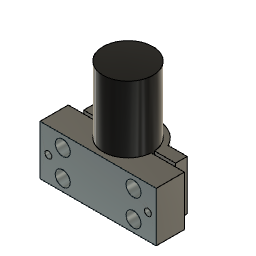
back_holder_thick (Autodesk Fusion 360 design; units mm, degrees)
Autodesk Fusion 360 part; units mm, degrees
note: some values were not read from the file. Set by a fixed rule: which sketch regions a step uses.
sketch "Sketch1" plane through (0, 0, 0) normal (0, 0, 1) x (1, 0, 0) in component "Pipe"
  circle A0 centre (0, 0) radius 15
  dimension "d1" = 30
  constraint coincident A0.centre origin
  measures "d1" diameter of A0
extrude "Extrude1" add sketch "Sketch1" along normal blind 70 makes body 1 in component "Pipe"
sketch "Sketch1 (2)" plane through (0, 0, 0) normal (0, 0, 1) x (1, 0, 0) in component "holder_under"
  circle A0 centre (0, 0) radius 15
  circle A1 centre (0, 0) radius 18
  line L0 (-17.9722, 1) -> (-27.6886, 1)
  line L1 (-27.6886, 1) -> (-27.6886, 8)
  line L2 (-27.6886, 8) -> (-12.6886, 8)
  line L3 (0, 0) -> (0, 15) construction
  line L4 (27.6886, 8) -> (12.6886, 8)
  line L5 (27.6886, 1) -> (27.6886, 8)
  line L6 (17.9722, 1) -> (27.6886, 1)
  line L7 (-17.9722, 1) -> (-14.9666, 1)
  line L8 (17.9722, 1) -> (14.9666, 1)
  dimension "d4" = 3
  dimension "d5" = 7
  dimension "d6" = 15
  dimension "d7" = 1
  constraint coincident A1 L0.start
  constraint horizontal L0
  constraint perpendicular L0 L1
  constraint coincident A0 L2.end
  constraint perpendicular L1 L2
  constraint coincident A0.centre A1.centre
  constraint coincident A0 L3.end
  constraint vertical L3
  constraint symmetric L0.start L3 L6.start
  constraint symmetric L0.end L3 L5.start
  constraint symmetric L1.end L3 L4.start
  constraint symmetric L2.end L3 L4.end
  constraint coincident A0 L7.end
  constraint parallel L0 L7
  constraint coincident A0 L8.end
  constraint parallel L6 L8
  measures "d5" distance of L0.end L1.end
  measures "d6" distance of L1.end L2.end
  measures "d7" distance of A0.centre L0
extrude "Extrude1'" add sketch "Sketch1 (2)" along normal blind 30 separate body contours A0 A1 L4 L8 | A0 A1 L2 L7 | A0 A1 L2 L4 | A1 L4 L5 L6 | A1 L0 L1 L2 makes body 2 in component "holder_under"
sketch "Sketch2" plane through (0, 1, 0) normal (0, -1, 0) x (1, 0, 0) in component "holder_under"
  line L0 (14.9666, 0) -> (27.6886, 0)
  line L1 (27.6886, 0) -> (27.6886, 30)
  line L2 (27.6886, 30) -> (14.9666, 30)
  line L3 (14.9666, 30) -> (14.9666, 0)
  line L4 (-21.3276, 30) -> (-21.3276, 0) construction
  line L5 (-27.6886, 30) -> (-14.9666, 30)
  line L6 (-14.9666, 0) -> (-27.6886, 0)
  line L7 (0, 0) -> (0, 30) construction
  line L8 (-14.9666, 30) -> (14.9666, 30)
  circle A0 centre (-21.3276, 23) radius 2.075
  circle A1 centre (-21.3276, 7) radius 2.075
  circle A2 centre (21.3276, 23) radius 2.075
  circle A3 centre (21.3276, 7) radius 2.075
  dimension "d10" = 4.15
  dimension "d11" = 4.15
  dimension "d12" = 7
  dimension "d13" = 7
  constraint vertical L4
  constraint coincident L4.start L5
  constraint coincident L4.end L6
  constraint midpoint L4.start L5
  constraint coincident L7.start origin
  constraint perpendicular L5 L7
  constraint coincident L7.end L8
  constraint coincident L4 A0.centre
  constraint coincident L4 A1.centre
  constraint symmetric L7 A0 A2
  constraint symmetric L7 A1 A3
  measures "d10" diameter of A0
  measures "d11" diameter of A1
  measures "d12" distance of L6 A1.centre
  measures "d13" distance of L5 A0.centre
extrude "Extrude2" cut sketch "Sketch2" against normal up to surface (7 mm away) contours A0 | A1 | A2 | A3 bodies 2 in component "holder_under"
sketch "Sketch1 (3)" plane through (0, 0, 0) normal (0, 0, 1) x (1, 0, 0) in component "holder_top"
  circle A0 centre (0, 0) radius 15
  circle A1 centre (0, 0) radius 18
  line L0 (-17.9722, -1) -> (-35, -1)
  line L1 (-35, -1) -> (-35, -18)
  line L2 (-35, -18) -> (0, -18)
  line L3 (0, 0) -> (0, -18) construction
  line L4 (35, -1) -> (35, -18)
  line L5 (35, -18) -> (0, -18)
  line L6 (17.9722, -1) -> (35, -1)
  line L7 (17.9722, -1) -> (14.9666, -1)
  line L8 (-17.9722, -1) -> (-14.9666, -1)
  dimension "d16" = 3
  dimension "d17" = 1
  dimension "d18" = 35
  constraint coincident A1 L0.start
  constraint horizontal L0
  constraint perpendicular L0 L1
  constraint perpendicular L1 L2
  constraint coincident A1 L2.end
  constraint tangent A1 L2
  constraint coincident A0.centre A1.centre
  constraint symmetric L0.start L3 L6.start
  constraint symmetric L0.end L3 L4.start
  constraint symmetric L1.end L3 L4.end
  constraint symmetric L2.end L3 L5.end
  constraint coincident A0 L7.end
  constraint parallel L6 L7
  constraint coincident A0 L8.end
  constraint parallel L0 L8
  measures "d17" distance of A0.centre L0
  measures "d18" distance of L1.end L2.end
extrude "Extrude1''" add sketch "Sketch1 (3)" along normal up to surface (30 mm away) separate body contours A0 A1 L7 L8 | A1 L0 L1 L2 | A1 L4 L5 L6 picked at (-1.1817, -16.9303) makes body 3 in component "holder_top"
sketch "Sketch2 (2)" plane through (0, -1, 0) normal (0, 1, 0) x (-1, 0, 0) in component "holder_top"
  line L0 (-14.9666, 30) -> (-35, 30)
  line L1 (-35, 30) -> (-35, 0)
  line L2 (-35, 0) -> (-14.9666, 0)
  line L3 (-14.9666, 0) -> (-14.9666, 30)
  circle A0 centre (-21.3276, 23) radius 2.075
  circle A1 centre (-21.3276, 7) radius 2.075
  circle A2 centre (21.3276, 7) radius 2.075
  circle A3 centre (21.3276, 23) radius 2.075
extrude "Extrude2'" cut sketch "Sketch2 (2)" against normal up to surface (17 mm away) contours A0 | A1 | A2 | A3 bodies 3 in component "holder_top"
sketch "Sketch3" plane through (0, 8, 0) normal (0, 1, 0) x (-1, 0, 0) in component "holder_under"
  circle A0 centre (21.3276, 7) radius 2.075
  circle A1 centre (21.3276, 23) radius 2.075
  line L0 (16.1245, 0) -> (27.6886, 0)
  line L1 (27.6886, 0) -> (27.6886, 30)
  line L2 (27.6886, 30) -> (16.1245, 30)
  line L3 (16.1245, 30) -> (16.1245, 0)
  line L4 (23.4061, 19.4) -> (25.4845, 23)
  line L5 (25.4845, 23) -> (23.4061, 26.6)
  line L6 (23.4061, 26.6) -> (19.2491, 26.6)
  line L7 (19.2491, 26.6) -> (17.1707, 23)
  line L8 (17.1707, 23) -> (19.2491, 19.4)
  line L9 (19.2491, 19.4) -> (23.4061, 19.4)
  line L10 (19.2491, 10.6) -> (17.1707, 7)
  line L11 (17.1707, 7) -> (19.2491, 3.4)
  line L12 (19.2491, 3.4) -> (23.4061, 3.4)
  line L13 (23.4061, 3.4) -> (25.4845, 7)
  line L14 (25.4845, 7) -> (23.4061, 10.6)
  line L15 (23.4061, 10.6) -> (19.2491, 10.6)
  line L16 (0, 0) -> (0, 30) construction
  line L17 (16.1245, 30) -> (-16.1245, 30)
  line L18 (-19.2491, 19.4) -> (-23.4061, 19.4)
  line L19 (-23.4061, 3.4) -> (-25.4845, 7)
  line L20 (-25.4845, 23) -> (-23.4061, 26.6)
  line L21 (-25.4845, 7) -> (-23.4061, 10.6)
  circle A2 centre (-21.3276, 7) radius 2.075
  circle A3 centre (-21.3276, 23) radius 2.075
  line L22 (-23.4061, 19.4) -> (-25.4845, 23)
  line L23 (-19.2491, 10.6) -> (-17.1707, 7)
  line L24 (-19.2491, 26.6) -> (-17.1707, 23)
  line L25 (-17.1707, 7) -> (-19.2491, 3.4)
  line L26 (-23.4061, 26.6) -> (-19.2491, 26.6)
  line L27 (-23.4061, 10.6) -> (-19.2491, 10.6)
  line L28 (-17.1707, 23) -> (-19.2491, 19.4)
  line L29 (-19.2491, 3.4) -> (-23.4061, 3.4)
  point P0 (21.3276, 23)
  point P1 (21.3276, 7)
  point P2 (-21.3276, 23)
  point P3 (-21.3276, 7)
  dimension "d23" = 7.2
  dimension "d24" = 7.2
  constraint coincident P0 A1.centre
  constraint coincident A0.centre P1
  constraint coincident L16.start origin
  constraint vertical L16
  constraint coincident L16.end L17
  constraint parallel L2 L12
  constraint parallel L2 L6
  constraint symmetric A0 L16 A2
  constraint symmetric A1 L16 A3
  constraint symmetric L4.start L16 L18.end
  constraint symmetric L4.end L16 L20.start
  constraint symmetric L5.end L16 L20.end
  constraint symmetric L6.end L16 L24.start
  constraint symmetric L7.end L16 L24.end
  constraint symmetric L8.end L16 L18.start
  constraint symmetric P0 L16 P2
  constraint symmetric L10.start L16 L23.start
  constraint symmetric L10.end L16 L23.end
  constraint symmetric L11.end L16 L25.end
  constraint symmetric L12.end L16 L19.start
  constraint symmetric L13.end L16 L19.end
  constraint symmetric L14.end L16 L21.end
  constraint symmetric P1 L16 P3
  measures "d23" distance of L4 L7
  measures "d24" distance of L10 L13
extrude "Extrude3" cut sketch "Sketch3" against normal blind 3 contours L4 L5 L6 L7 L8 L9 | L10 L11 L12 L13 L14 L15 | L18 L20 L22 L24 L26 L28 | L19 L21 L23 L25 L27 L29 bodies 2 in component "holder_under"
sketch "Sketch3 (2)" plane through (0, -18, 0) normal (0, -1, 0) x (1, 0, 0) in component "holder_top"
  circle A0 centre (21.3276, 7) radius 2.075
  circle A1 centre (-21.3276, 7) radius 2.075
  circle A2 centre (21.3276, 23) radius 2.075
  circle A3 centre (-21.3276, 23) radius 2.075
  line L0 (35, 30) -> (-35, 30)
  line L1 (-35, 30) -> (-35, 0)
  line L2 (-35, 0) -> (35, 0)
  line L3 (35, 0) -> (35, 30)
  circle A4 centre (-21.3276, 23) radius 4.5
  circle A5 centre (-21.3276, 7) radius 4.5
  circle A6 centre (21.3276, 7) radius 4.5
  circle A7 centre (21.3276, 23) radius 4.5
  dimension "d27" = 9
  dimension "d28" = 9
  dimension "d29" = 9
  dimension "d30" = 9
  constraint concentric A3 A4
  constraint concentric A1 A5
  constraint concentric A0 A6
  constraint concentric A2 A7
  measures "d27" diameter of A4
  measures "d28" diameter of A5
  measures "d29" diameter of A6
  measures "d30" diameter of A7
extrude "Extrude3'" cut sketch "Sketch3 (2)" against normal up to surface (13 mm away) contours A4 | A5 | A6 | A7 bodies 3 in component "holder_top"
sketch "Sketch1 (4)" plane through (0, -18, 0) normal (0, -1, 0) x (1, 0, 0)
  circle A0 centre (-21.3276, 7) radius 4.5
  circle A1 centre (21.3276, 7) radius 4.5
  circle A2 centre (-21.3276, 23) radius 4.5
  circle A3 centre (21.3276, 23) radius 4.5
  line L0 (35, 30) -> (-35, 30)
  line L1 (-35, 30) -> (-35, 0)
  line L2 (-35, 0) -> (35, 0)
  line L3 (35, 0) -> (35, 30)
sketch "Sketch4" plane through (0, -18, 15) normal (0, -1, 0) x (1, 0, 0) in component "holder_top"
  line L0 (0, 0) -> (-35, 0) construction
  line L1 (-35, 15) -> (-35, -15)
  line L2 (0, 0) -> (0, 15) construction
  circle A0 centre (-30, 0) radius 2.075
  line L3 (35, 15) -> (-35, 15)
  circle A1 centre (30, 0) radius 2.075
  dimension "d33" = 4.15
  dimension "d34" = 5
  constraint coincident L0.start L2.start
  constraint horizontal L0
  constraint coincident L0.end L1
  constraint perpendicular L0 L2
  constraint coincident L0 A0.centre
  constraint coincident L2.end L3
  constraint symmetric L2 A0 A1
  measures "d33" diameter of A0
  measures "d34" distance of L0.end A0.centre
extrude "Extrude4" cut sketch "Sketch4" against normal up to surface (17 mm away) bodies 3 in component "holder_top"
sketch "Sketch5" plane through (0, -1, 0) normal (0, 1, 0) x (-1, 0, 0) in component "holder_top"
  circle A0 centre (-30, 15) radius 2.075
  circle A1 centre (-21.3276, 7) radius 2.075
  circle A2 centre (-21.3276, 23) radius 2.075
  line L0 (-14.9666, 30) -> (-35, 30)
  line L1 (-35, 30) -> (-35, 0)
  line L2 (-35, 0) -> (-14.9666, 0)
  line L3 (-14.9666, 0) -> (-14.9666, 30)
  line L4 (-30, 19.0415) -> (-33.5, 17.0207)
  line L5 (-33.5, 17.0207) -> (-33.5, 12.9793)
  line L6 (-33.5, 12.9793) -> (-30, 10.9585)
  line L7 (-30, 10.9585) -> (-26.5, 12.9793)
  line L8 (-26.5, 12.9793) -> (-26.5, 17.0207)
  line L9 (-26.5, 17.0207) -> (-30, 19.0415)
  line L10 (0, 0) -> (0, 30) construction
  line L11 (-35, 30) -> (35, 30)
  line L12 (26.5, 17.0207) -> (30, 19.0415)
  line L13 (30, 19.0415) -> (33.5, 17.0207)
  line L14 (33.5, 17.0207) -> (33.5, 12.9793)
  line L15 (33.5, 12.9793) -> (30, 10.9585)
  line L16 (30, 10.9585) -> (26.5, 12.9793)
  line L17 (26.5, 12.9793) -> (26.5, 17.0207)
  point P0 (-30, 15)
  dimension "d40" = 7
  constraint coincident P0 A0.centre
  constraint coincident L10.start origin
  constraint vertical L10
  constraint coincident L10.end L11
  constraint parallel L1 L5
  constraint symmetric L4.start L10 L12.end
  constraint symmetric L4.end L10 L13.end
  constraint symmetric L5.end L10 L14.end
  constraint symmetric L6.end L10 L15.end
  constraint symmetric L7.end L10 L16.end
  constraint symmetric L8.end L10 L12.start
  measures "d40" distance of L5 L8
extrude "Extrude5" cut sketch "Sketch5" against normal blind 6 contours L4 L5 L6 L7 L8 L9 | L12 L13 L14 L15 L16 L17 bodies 3 in component "holder_top"
component "Pipe" placed x (1, 0, 0) y (0, 1, 0) z (0, 0, 1) at (0, 0, 0)
component "holder_under" placed x (1, 0, 0) y (0, 1, 0) z (0, 0, 1) at (0, 0, 0)
component "holder_top" placed x (1, 0, 0) y (0, 1, 0) z (0, 0, 1) at (0, 0, 0)
